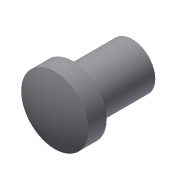
# Autodesk Inventor part: 100_CCTV_Fisheye_Starlight_f2.8mm_Fno_1.4
Saved by Autodesk Inventor 2019 (Build 230136000, 136)
## iProperties
Created: 2019-06-17
Part Number: 100_CCTV_Fisheye_Starlight_f2.8mm_Fno_1.4
Material: Generic
Document SubType Name: Modeling
Designer: diederichbenedict
Density: 1 g/cm^3
Appearance: Default
Author: diederichbenedict
Autodesk Inventor part; units mm, degrees
ref_plane "YZ Plane" through (0, 0, 0) normal (1, 0, 0) x (0, 1, 0)
ref_plane "XZ Plane" through (0, 0, 0) normal (0, 1, 0) x (-1, 0, 0)
ref_plane "XY Plane" through (0, 0, 0) normal (0, 0, 1) x (1, 0, 0)
sketch "Sketch1" plane through (0, 0, 0) normal (1, 0, 0) x (0, 1, 0)
  line L0 (0, 0) -> (0, -20.1)
  line L1 (0, -20.1) -> (-6, -20.1)
  line L2 (-6, -20.1) -> (-6, -4.7)
  line L3 (-6, -4.7) -> (-8.75, -4.7)
  line L4 (-8.75, -4.7) -> (-8.75, 0)
  arc A0 (0, 1.822) -> (-8.75, 0) centre (0, -20.1) ccw
  line L5 (0, 1.822) -> (0, 0)
  dimension "d0" = 20.1
  dimension "d1" = 6
  dimension "d2" = 15.4
  dimension "d3" = 8.75
  dimension "d4" = 0
  constraints: 12 end point, 3 perpendicular, 2 point on circle, 1 centre point, 1 coincident, 1 collinear, 1 horizontal, 1 vertical
  measures "d0" distance of L0.start L0.end
  measures "d1" distance of L0.end L1.end
  measures "d2" distance of L1.end L2.end
  measures "d3" distance between parallel lines of L0 L4
  measures "d4" vertical distance of L0.start L4.end
revolve "Revolution1" add sketch "Sketch1" angle 360 about axis through (0, 0, 0) along (0, 0, -1)
body "Solid1"
